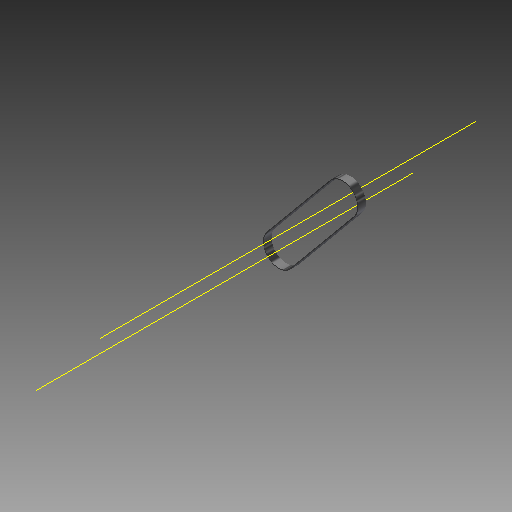
# Autodesk Inventor part: Synchronous Belt
Saved by Autodesk Inventor 2019.4 (Build 234330000, 330)
## iProperties
Created: 2019-11-30
Part Number: Synchronous Belt
Material: Rubber
Document SubType Name: Modeling
Designer: admin
Density: 0.93 g/cm^3
Appearance: Rubber - Black - Version 1.1
Mass: 1.2834 g
Surface Area: 48.76 cm^2
Volume: 1.38 cm^3
CustomPartVersion: 1
Author: admin
Autodesk Inventor part; units mm, degrees
sketch "Sketch Path" plane through (0, 0, 0) normal (0, 0, 1) x (1, 0, 0)
  arc A0 (-9.1902, 7.6173) -> (9.1902, -7.6173) centre (0, 0) ccw
  arc A1 (58.6465, 52.0512) -> (40.2661, 67.2858) centre (49.4563, 59.6685) ccw
  line L0 (58.6465, 52.0512) -> (9.1902, -7.6173)
  line L1 (-9.1902, 7.6173) -> (40.2661, 67.2858)
  constraints: 4 end point, 4 point on circle, 2 centre point
ref_plane "Cross Section Plane" through (9.1902, -7.6173, 0) normal (0.6381, 0.7699, 0) x (0, 0, 1)
ref_plane "Work Plane2" through (0, 0, 0) normal (-1, 0, 0) x (0, 0, 1)
ref_plane "Work Plane3" through (49.4563, 59.6685, 0) normal (-0.6691, -0.7431, 0) x (0, 0, 1)
sketch "Cross Section" plane through (9.1902, -7.6173, 0) normal (0.6381, 0.7699, 0) x (0, 0, 1)
  line L0 (-3, 0.3) -> (3, 0.3)
  line L1 (3, 0.3) -> (3, -0.3)
  line L2 (3, -0.3) -> (-3, -0.3)
  line L3 (-3, -0.3) -> (-3, 0.3)
  line L4 (-3, 0) -> (3, 0) construction
  point P0 (0, 0)
  point P1 (0, 0)
  dimension "d0" = 6
  dimension "d4" = 0.3
  dimension "d5" = 0.3
  constraints: 10 end point, 3 midpoint, 2 parallel, 1 coincident, 1 horizontal, 1 perpendicular, 1 other
  measures "d0" distance between parallel lines of L1 L3
  measures "d4" distance between parallel lines of L2 L4
  measures "d5" distance between parallel lines of L4 L0
sweep "Belt" add profiles "Cross Section" path "Sketch Path"
equation "\"d0\" = da_B"
equation "\"d4\" = da_a"
equation "\"d5\" = da_a2"
equation "\"da_B\" = 6"
equation "\"da_pb\" = 2.5"
equation "\"da_a\" = 0.3"
equation "\"da_S\" = 1.5"
equation "\"da_Beta\" = 20deg"
equation "\"da_Ht\" = 0.7"
equation "\"da_H\" = 1.3"
equation "\"da_a2\" = 0.3"
body "Solid1"
